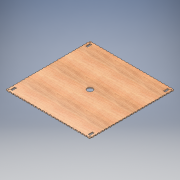
# Autodesk Inventor part: КВ33.044.002 - Дно блока управления
Saved by Autodesk Inventor 2019 (Build 230136000, 136)
## iProperties
Created: 2019-08-10
Part Number: КВ33.044.002 - Дно блока управления
Material: Дерево (береза)
Document SubType Name: Modeling
Designer: Петров Иван
Density: 0.55 g/cm^3
Appearance: Береза — натуральный — полированный
Author: Петров Иван
Autodesk Inventor part; units mm, degrees
ref_plane "YZ Plane" through (0, 0, 0) normal (1, 0, 0) x (0, 1, 0)
ref_plane "XZ Plane" through (0, 0, 0) normal (0, 1, 0) x (-1, 0, 0)
ref_plane "XY Plane" through (0, 0, 0) normal (0, 0, 1) x (1, 0, 0)
sketch "Эскиз1" plane through (0, 0, 0) normal (0, 1, 0) x (-1, 0, 0)
  line L0 (-367, 367) -> (367, 367)
  line L1 (367, 367) -> (367, -367)
  line L2 (367, -367) -> (-367, -367)
  line L3 (-367, -367) -> (-367, 367)
  line L4 (-367, 367) -> (367, -367) construction
  line L5 (367, 367) -> (-367, -367) construction
  point P0 (0, 0)
  dimension "d0" = 734
  dimension "d1" = 734
  constraints: 12 end point, 2 midpoint, 2 parallel, 1 horizontal, 1 perpendicular
  measures "d0" distance of L1.end L2.end
  measures "d1" distance of L0.end L1.end
extrude "Выдавливание1" add sketch "Эскиз1" along normal blind 8
sketch "Эскиз3" plane through (0, 8, 0) normal (0, 1, 0) x (1, 0, 0)
  line L0 (-367, 367) -> (-367, -367) projected
  line L1 (-367, -367) -> (-370, -367)
  line L2 (-370, -367) -> (-370, -351)
  line L3 (-370, -351) -> (-367, -351)
  line L4 (-367, -351) -> (-367, -367)
  line L5 (-367, -335) -> (-370, -335)
  line L6 (-370, -335) -> (-370, -319)
  line L7 (-370, -319) -> (-367, -319)
  line L8 (-367, -319) -> (-367, -335)
  line L9 (-367, -303) -> (-370, -303)
  line L10 (-370, -303) -> (-370, -287)
  line L11 (-370, -287) -> (-367, -287)
  line L12 (-367, -287) -> (-367, -303)
  line L13 (-367, -271) -> (-370, -271)
  line L14 (-370, -271) -> (-370, -255)
  line L15 (-370, -255) -> (-367, -255)
  line L16 (-367, -255) -> (-367, -271)
  line L17 (-367, -239) -> (-370, -239)
  line L18 (-370, -239) -> (-370, -223)
  line L19 (-370, -223) -> (-367, -223)
  line L20 (-367, -223) -> (-367, -239)
  line L21 (-367, -207) -> (-370, -207)
  line L22 (-370, -207) -> (-370, -191)
  line L23 (-370, -191) -> (-367, -191)
  line L24 (-367, -191) -> (-367, -207)
  line L25 (-367, -175) -> (-370, -175)
  line L26 (-370, -175) -> (-370, -159)
  line L27 (-370, -159) -> (-367, -159)
  line L28 (-367, -159) -> (-367, -175)
  line L29 (-367, -143) -> (-370, -143)
  line L30 (-370, -143) -> (-370, -127)
  line L31 (-370, -127) -> (-367, -127)
  line L32 (-367, -127) -> (-367, -143)
  line L33 (-367, -111) -> (-370, -111)
  line L34 (-370, -111) -> (-370, -95)
  line L35 (-370, -95) -> (-367, -95)
  line L36 (-367, -95) -> (-367, -111)
  line L37 (-367, -79) -> (-370, -79)
  line L38 (-370, -79) -> (-370, -63)
  line L39 (-370, -63) -> (-367, -63)
  line L40 (-367, -63) -> (-367, -79)
  line L41 (-367, -47) -> (-370, -47)
  line L42 (-370, -47) -> (-370, -31)
  line L43 (-370, -31) -> (-367, -31)
  line L44 (-367, -31) -> (-367, -47)
  line L45 (-367, -15) -> (-370, -15)
  line L46 (-370, -15) -> (-370, 1)
  line L47 (-370, 1) -> (-367, 1)
  line L48 (-367, 1) -> (-367, -15)
  line L49 (-367, 17) -> (-370, 17)
  line L50 (-370, 17) -> (-370, 33)
  line L51 (-370, 33) -> (-367, 33)
  line L52 (-367, 33) -> (-367, 17)
  line L53 (-367, 49) -> (-370, 49)
  line L54 (-370, 49) -> (-370, 65)
  line L55 (-370, 65) -> (-367, 65)
  line L56 (-367, 65) -> (-367, 49)
  line L57 (-367, 81) -> (-370, 81)
  line L58 (-370, 81) -> (-370, 97)
  line L59 (-370, 97) -> (-367, 97)
  line L60 (-367, 97) -> (-367, 81)
  line L61 (-367, 113) -> (-370, 113)
  line L62 (-370, 113) -> (-370, 129)
  line L63 (-370, 129) -> (-367, 129)
  line L64 (-367, 129) -> (-367, 113)
  line L65 (-367, 145) -> (-370, 145)
  line L66 (-370, 145) -> (-370, 161)
  line L67 (-370, 161) -> (-367, 161)
  line L68 (-367, 161) -> (-367, 145)
  line L69 (-367, 177) -> (-370, 177)
  line L70 (-370, 177) -> (-370, 193)
  line L71 (-370, 193) -> (-367, 193)
  line L72 (-367, 193) -> (-367, 177)
  line L73 (-367, 209) -> (-370, 209)
  line L74 (-370, 209) -> (-370, 225)
  line L75 (-370, 225) -> (-367, 225)
  line L76 (-367, 225) -> (-367, 209)
  line L77 (-367, 241) -> (-370, 241)
  line L78 (-370, 241) -> (-370, 257)
  line L79 (-370, 257) -> (-367, 257)
  line L80 (-367, 257) -> (-367, 241)
  line L81 (-367, 273) -> (-370, 273)
  line L82 (-370, 273) -> (-370, 289)
  line L83 (-370, 289) -> (-367, 289)
  line L84 (-367, 289) -> (-367, 273)
  line L85 (-367, 305) -> (-370, 305)
  line L86 (-370, 305) -> (-370, 321)
  line L87 (-370, 321) -> (-367, 321)
  line L88 (-367, 321) -> (-367, 305)
  line L89 (-367, 337) -> (-370, 337)
  line L90 (-370, 337) -> (-370, 353)
  line L91 (-370, 353) -> (-367, 353)
  line L92 (-367, 353) -> (-367, 337)
  line L93 (-367, 367) -> (-351, 367)
  line L94 (-351, 367) -> (-351, 370)
  line L95 (-351, 370) -> (-367, 370)
  line L96 (-367, 370) -> (-367, 367)
  line L97 (-335, 370) -> (-335, 367)
  line L98 (-319, 367) -> (-319, 370)
  line L99 (-319, 370) -> (-335, 370)
  line L100 (-335, 367) -> (-319, 367)
  line L101 (-303, 370) -> (-303, 367)
  line L102 (-287, 367) -> (-287, 370)
  line L103 (-287, 370) -> (-303, 370)
  line L104 (-303, 367) -> (-287, 367)
  line L105 (-271, 370) -> (-271, 367)
  line L106 (-255, 367) -> (-255, 370)
  line L107 (-255, 370) -> (-271, 370)
  line L108 (-271, 367) -> (-255, 367)
  line L109 (-239, 370) -> (-239, 367)
  line L110 (-223, 367) -> (-223, 370)
  line L111 (-223, 370) -> (-239, 370)
  line L112 (-239, 367) -> (-223, 367)
  line L113 (-207, 370) -> (-207, 367)
  line L114 (-191, 367) -> (-191, 370)
  line L115 (-191, 370) -> (-207, 370)
  line L116 (-207, 367) -> (-191, 367)
  line L117 (-175, 370) -> (-175, 367)
  line L118 (-159, 367) -> (-159, 370)
  line L119 (-159, 370) -> (-175, 370)
  line L120 (-175, 367) -> (-159, 367)
  line L121 (-143, 370) -> (-143, 367)
  line L122 (-127, 367) -> (-127, 370)
  line L123 (-127, 370) -> (-143, 370)
  line L124 (-143, 367) -> (-127, 367)
  line L125 (-111, 370) -> (-111, 367)
  line L126 (-95, 367) -> (-95, 370)
  line L127 (-95, 370) -> (-111, 370)
  line L128 (-111, 367) -> (-95, 367)
  line L129 (-79, 370) -> (-79, 367)
  line L130 (-63, 367) -> (-63, 370)
  line L131 (-63, 370) -> (-79, 370)
  line L132 (-79, 367) -> (-63, 367)
  line L133 (-47, 370) -> (-47, 367)
  line L134 (-31, 367) -> (-31, 370)
  line L135 (-31, 370) -> (-47, 370)
  line L136 (-47, 367) -> (-31, 367)
  line L137 (-15, 370) -> (-15, 367)
  line L138 (1, 367) -> (1, 370)
  line L139 (1, 370) -> (-15, 370)
  line L140 (-15, 367) -> (1, 367)
  line L141 (17, 370) -> (17, 367)
  line L142 (33, 367) -> (33, 370)
  line L143 (33, 370) -> (17, 370)
  line L144 (17, 367) -> (33, 367)
  line L145 (49, 370) -> (49, 367)
  line L146 (65, 367) -> (65, 370)
  line L147 (65, 370) -> (49, 370)
  line L148 (49, 367) -> (65, 367)
  line L149 (81, 370) -> (81, 367)
  line L150 (97, 367) -> (97, 370)
  line L151 (97, 370) -> (81, 370)
  line L152 (81, 367) -> (97, 367)
  line L153 (113, 370) -> (113, 367)
  line L154 (129, 367) -> (129, 370)
  line L155 (129, 370) -> (113, 370)
  line L156 (113, 367) -> (129, 367)
  line L157 (145, 370) -> (145, 367)
  line L158 (161, 367) -> (161, 370)
  line L159 (161, 370) -> (145, 370)
  line L160 (145, 367) -> (161, 367)
  line L161 (177, 370) -> (177, 367)
  line L162 (193, 367) -> (193, 370)
  line L163 (193, 370) -> (177, 370)
  line L164 (177, 367) -> (193, 367)
  line L165 (209, 370) -> (209, 367)
  line L166 (225, 367) -> (225, 370)
  line L167 (225, 370) -> (209, 370)
  line L168 (209, 367) -> (225, 367)
  line L169 (241, 370) -> (241, 367)
  line L170 (257, 367) -> (257, 370)
  line L171 (257, 370) -> (241, 370)
  line L172 (241, 367) -> (257, 367)
  line L173 (273, 370) -> (273, 367)
  line L174 (289, 367) -> (289, 370)
  line L175 (289, 370) -> (273, 370)
  line L176 (273, 367) -> (289, 367)
  line L177 (305, 370) -> (305, 367)
  line L178 (321, 367) -> (321, 370)
  line L179 (321, 370) -> (305, 370)
  line L180 (305, 367) -> (321, 367)
  line L181 (337, 370) -> (337, 367)
  line L182 (353, 367) -> (353, 370)
  line L183 (353, 370) -> (337, 370)
  line L184 (337, 367) -> (353, 367)
  line L185 (367, -367) -> (367, 367) projected
  line L186 (367, 367) -> (370, 367)
  line L187 (370, 367) -> (370, 351)
  line L188 (370, 351) -> (367, 351)
  line L189 (367, 351) -> (367, 367)
  line L190 (367, 319) -> (367, 335)
  line L191 (367, 335) -> (370, 335)
  line L192 (370, 335) -> (370, 319)
  line L193 (370, 319) -> (367, 319)
  line L194 (367, 287) -> (367, 303)
  line L195 (367, 303) -> (370, 303)
  line L196 (370, 303) -> (370, 287)
  line L197 (370, 287) -> (367, 287)
  line L198 (367, 255) -> (367, 271)
  line L199 (367, 271) -> (370, 271)
  line L200 (370, 271) -> (370, 255)
  line L201 (370, 255) -> (367, 255)
  line L202 (367, 223) -> (367, 239)
  line L203 (367, 239) -> (370, 239)
  line L204 (370, 239) -> (370, 223)
  line L205 (370, 223) -> (367, 223)
  line L206 (367, 191) -> (367, 207)
  line L207 (367, 207) -> (370, 207)
  line L208 (370, 207) -> (370, 191)
  line L209 (370, 191) -> (367, 191)
  line L210 (367, 159) -> (367, 175)
  line L211 (367, 175) -> (370, 175)
  line L212 (370, 175) -> (370, 159)
  line L213 (370, 159) -> (367, 159)
  line L214 (367, 127) -> (367, 143)
  line L215 (367, 143) -> (370, 143)
  line L216 (370, 143) -> (370, 127)
  line L217 (370, 127) -> (367, 127)
  line L218 (367, 95) -> (367, 111)
  line L219 (367, 111) -> (370, 111)
  line L220 (370, 111) -> (370, 95)
  line L221 (370, 95) -> (367, 95)
  line L222 (367, 63) -> (367, 79)
  line L223 (367, 79) -> (370, 79)
  line L224 (370, 79) -> (370, 63)
  line L225 (370, 63) -> (367, 63)
  line L226 (367, 31) -> (367, 47)
  line L227 (367, 47) -> (370, 47)
  line L228 (370, 47) -> (370, 31)
  line L229 (370, 31) -> (367, 31)
  line L230 (367, -1) -> (367, 15)
  line L231 (367, 15) -> (370, 15)
  line L232 (370, 15) -> (370, -1)
  line L233 (370, -1) -> (367, -1)
  line L234 (367, -33) -> (367, -17)
  line L235 (367, -17) -> (370, -17)
  line L236 (370, -17) -> (370, -33)
  line L237 (370, -33) -> (367, -33)
  line L238 (367, -65) -> (367, -49)
  line L239 (367, -49) -> (370, -49)
  line L240 (370, -49) -> (370, -65)
  line L241 (370, -65) -> (367, -65)
  line L242 (367, -97) -> (367, -81)
  line L243 (367, -81) -> (370, -81)
  line L244 (370, -81) -> (370, -97)
  line L245 (370, -97) -> (367, -97)
  line L246 (367, -129) -> (367, -113)
  line L247 (367, -113) -> (370, -113)
  line L248 (370, -113) -> (370, -129)
  line L249 (370, -129) -> (367, -129)
  line L250 (367, -161) -> (367, -145)
  line L251 (367, -145) -> (370, -145)
  line L252 (370, -145) -> (370, -161)
  line L253 (370, -161) -> (367, -161)
  line L254 (367, -193) -> (367, -177)
  line L255 (367, -177) -> (370, -177)
  line L256 (370, -177) -> (370, -193)
  line L257 (370, -193) -> (367, -193)
  line L258 (367, -225) -> (367, -209)
  line L259 (367, -209) -> (370, -209)
  line L260 (370, -209) -> (370, -225)
  line L261 (370, -225) -> (367, -225)
  line L262 (367, -257) -> (367, -241)
  line L263 (367, -241) -> (370, -241)
  line L264 (370, -241) -> (370, -257)
  line L265 (370, -257) -> (367, -257)
  line L266 (367, -289) -> (367, -273)
  line L267 (367, -273) -> (370, -273)
  line L268 (370, -273) -> (370, -289)
  line L269 (370, -289) -> (367, -289)
  line L270 (367, -321) -> (367, -305)
  line L271 (367, -305) -> (370, -305)
  line L272 (370, -305) -> (370, -321)
  line L273 (370, -321) -> (367, -321)
  line L274 (367, -353) -> (367, -337)
  line L275 (367, -337) -> (370, -337)
  line L276 (370, -337) -> (370, -353)
  line L277 (370, -353) -> (367, -353)
  line L278 (367, -367) -> (351, -367)
  line L279 (351, -367) -> (351, -370)
  line L280 (351, -370) -> (367, -370)
  line L281 (367, -370) -> (367, -367)
  line L282 (335, -367) -> (319, -367)
  line L283 (319, -367) -> (319, -370)
  line L284 (319, -370) -> (335, -370)
  line L285 (335, -370) -> (335, -367)
  line L286 (303, -367) -> (287, -367)
  line L287 (287, -367) -> (287, -370)
  line L288 (287, -370) -> (303, -370)
  line L289 (303, -370) -> (303, -367)
  line L290 (271, -367) -> (255, -367)
  line L291 (255, -367) -> (255, -370)
  line L292 (255, -370) -> (271, -370)
  line L293 (271, -370) -> (271, -367)
  line L294 (239, -367) -> (223, -367)
  line L295 (223, -367) -> (223, -370)
  line L296 (223, -370) -> (239, -370)
  line L297 (239, -370) -> (239, -367)
  line L298 (207, -367) -> (191, -367)
  line L299 (191, -367) -> (191, -370)
  line L300 (191, -370) -> (207, -370)
  line L301 (207, -370) -> (207, -367)
  line L302 (175, -367) -> (159, -367)
  line L303 (159, -367) -> (159, -370)
  line L304 (159, -370) -> (175, -370)
  line L305 (175, -370) -> (175, -367)
  line L306 (143, -367) -> (127, -367)
  line L307 (127, -367) -> (127, -370)
  line L308 (127, -370) -> (143, -370)
  line L309 (143, -370) -> (143, -367)
  line L310 (111, -367) -> (95, -367)
  line L311 (95, -367) -> (95, -370)
  line L312 (95, -370) -> (111, -370)
  line L313 (111, -370) -> (111, -367)
  line L314 (79, -367) -> (63, -367)
  line L315 (63, -367) -> (63, -370)
  line L316 (63, -370) -> (79, -370)
  line L317 (79, -370) -> (79, -367)
  line L318 (47, -367) -> (31, -367)
  line L319 (31, -367) -> (31, -370)
  line L320 (31, -370) -> (47, -370)
  line L321 (47, -370) -> (47, -367)
  line L322 (15, -367) -> (-1, -367)
  line L323 (-1, -367) -> (-1, -370)
  line L324 (-1, -370) -> (15, -370)
  line L325 (15, -370) -> (15, -367)
  line L326 (-17, -367) -> (-33, -367)
  line L327 (-33, -367) -> (-33, -370)
  line L328 (-33, -370) -> (-17, -370)
  line L329 (-17, -370) -> (-17, -367)
  line L330 (-49, -367) -> (-65, -367)
  line L331 (-65, -367) -> (-65, -370)
  line L332 (-65, -370) -> (-49, -370)
  line L333 (-49, -370) -> (-49, -367)
  line L334 (-81, -367) -> (-97, -367)
  line L335 (-97, -367) -> (-97, -370)
  line L336 (-97, -370) -> (-81, -370)
  line L337 (-81, -370) -> (-81, -367)
  line L338 (-113, -367) -> (-129, -367)
  line L339 (-129, -367) -> (-129, -370)
  line L340 (-129, -370) -> (-113, -370)
  line L341 (-113, -370) -> (-113, -367)
  line L342 (-145, -367) -> (-161, -367)
  line L343 (-161, -367) -> (-161, -370)
  line L344 (-161, -370) -> (-145, -370)
  line L345 (-145, -370) -> (-145, -367)
  line L346 (-177, -367) -> (-193, -367)
  line L347 (-193, -367) -> (-193, -370)
  line L348 (-193, -370) -> (-177, -370)
  line L349 (-177, -370) -> (-177, -367)
  line L350 (-209, -367) -> (-225, -367)
  line L351 (-225, -367) -> (-225, -370)
  line L352 (-225, -370) -> (-209, -370)
  line L353 (-209, -370) -> (-209, -367)
  line L354 (-241, -367) -> (-257, -367)
  line L355 (-257, -367) -> (-257, -370)
  line L356 (-257, -370) -> (-241, -370)
  line L357 (-241, -370) -> (-241, -367)
  line L358 (-273, -367) -> (-289, -367)
  line L359 (-289, -367) -> (-289, -370)
  line L360 (-289, -370) -> (-273, -370)
  line L361 (-273, -370) -> (-273, -367)
  line L362 (-305, -367) -> (-321, -367)
  line L363 (-321, -367) -> (-321, -370)
  line L364 (-321, -370) -> (-305, -370)
  line L365 (-305, -370) -> (-305, -367)
  line L366 (-337, -367) -> (-353, -367)
  line L367 (-353, -367) -> (-353, -370)
  line L368 (-353, -370) -> (-337, -370)
  line L369 (-337, -370) -> (-337, -367)
  point P0 (0, 0)
  dimension "d4" = 3
  dimension "d5" = 16
  dimension "d8" = 32
  dimension "d13" = 16
  dimension "d14" = 3
  dimension "d17" = 32
  dimension "d22" = 3
  dimension "d23" = 16
  dimension "d26" = 32
  dimension "d31" = 16
  dimension "d32" = 3
  dimension "d35" = 32
  constraints: 736 end point, 8 parallel, 6 horizontal, 4 perpendicular, 3 collinear, 2 vertical, 701 other
  measures "d4" distance of L2.end L3.end
  measures "d5" distance of L1.end L2.end
  measures "d8" distance of L2.end L6.end
  measures "d13" distance of L95.end L94.end
  measures "d14" distance of L94.end L93.end
  measures "d17" distance of L93.end L98.start
  measures "d22" distance of L187.end L188.end
  measures "d23" distance of L186.end L187.end
  measures "d26" distance of L188.end L190.start
  measures "d31" distance of L280.end L279.end
  measures "d32" distance of L279.end L278.end
  measures "d35" distance of L278.end L282.end
extrude "Выдавливание2" add sketch "Эскиз3" against normal blind 8
sketch "Эскиз4" plane through (0, 8, 0) normal (0, 1, 0) x (1, 0, 0)
  line L0 (305, 370) -> (321, 370) projected
  line L1 (313, 370) -> (313, 357.5)
  line L2 (370, 351) -> (370, 367) projected
  line L3 (370, 357.5) -> (313, 357.5)
  line L4 (370, 357.5) -> (357.5, 357.5)
  circle A0 centre (357.5, 357.5) radius 4.1
  line L5 (0, 0) -> (0, 59.4611)
  line L6 (0, 0) -> (-60.8866, 0)
  circle A1 centre (357.5, -357.5) radius 4.1
  circle A2 centre (-357.5, 357.5) radius 4.1
  circle A3 centre (-357.5, -357.5) radius 4.1
  dimension "d42" = 12.5
  dimension "d43" = 12.5
  dimension "d44" = 8.2
  constraints: 10 end point, 4 centre point, 3 symmetric about line, 2 point on line, 2 vertical, 1 coincident, 1 horizontal, 1 midpoint, 1 perpendicular, 3 other
  measures "d42" distance of L1.start L1.end
  measures "d43" distance of L3.start L4.end
  measures "d44" diameter of A0
extrude "Выдавливание3" cut sketch "Эскиз4" against normal blind 10
sketch "Эскиз6" plane through (0, 8, 0) normal (0, 1, 0) x (1, 0, 0)
  line L0 (-333.081, -350) -> (-350, -350)
  line L1 (-350, -350) -> (-350, -312.2438)
  line L2 (-350, -312.2438) -> (-333.081, -312.2438)
  line L3 (-333.081, -312.2438) -> (-333.081, -350)
  line L4 (-337, -370) -> (-353, -370) projected
  line L5 (-370, -319) -> (-370, -335) projected
  line L6 (0, 0) -> (0, 58.8513)
  line L7 (0, 0) -> (-73.7249, 0)
  line L8 (-333.081, 350) -> (-350, 350)
  line L9 (-350, 350) -> (-350, 312.2438)
  line L10 (-350, 312.2438) -> (-333.081, 312.2438)
  line L11 (-333.081, 312.2438) -> (-333.081, 350)
  line L12 (333.081, -350) -> (350, -350)
  line L13 (350, -350) -> (350, -312.2438)
  line L14 (350, -312.2438) -> (333.081, -312.2438)
  line L15 (333.081, -312.2438) -> (333.081, -350)
  line L16 (337, -370) -> (353, -370)
  line L17 (370, -319) -> (370, -335)
  line L18 (333.081, 350) -> (350, 350)
  line L19 (350, 350) -> (350, 312.2438)
  line L20 (350, 312.2438) -> (333.081, 312.2438)
  line L21 (333.081, 312.2438) -> (333.081, 350)
  dimension "d50" = 20
  dimension "d51" = 20
  constraints: 40 end point, 16 symmetric about line, 2 horizontal, 2 parallel, 1 perpendicular, 1 vertical
  measures "d50" distance between parallel lines of L4 L0
  measures "d51" distance between parallel lines of L1 L5
extrude "Выдавливание4" cut sketch "Эскиз6" against normal blind 10
sketch "Эскиз7" plane through (0, 8, 0) normal (0, 1, 0) x (1, 0, 0)
  circle A0 centre (0, 0) radius 25
  dimension "d54" = 50
  constraints: 1 centre point, 1 coincident
  measures "d54" diameter of A0
extrude "Выдавливание5" cut sketch "Эскиз7" against normal blind 10
